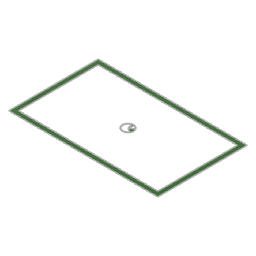
_car box.42bf6e30-fc25-4c0d-9044-dd2759e64512 (Autodesk Fusion 360 design; units mm, degrees)
Autodesk Fusion 360 part; units mm, degrees
sketch "Sketch1" plane through (0, 0, 0) normal (0, 0, 1) x (1, 0, 0)
  line L0 (-177.8, 101.6) -> (177.8, 101.6)
  line L1 (177.8, 101.6) -> (177.8, -101.6)
  line L2 (177.8, -101.6) -> (-177.8, -101.6)
  line L3 (-177.8, -101.6) -> (-177.8, 101.6)
  line L4 (-177.8, 101.6) -> (177.8, -101.6) construction
  line L5 (177.8, 101.6) -> (-177.8, -101.6) construction
  circle A0 centre (0, 0) radius 12.7
  line L6 (11.0267, -6.301) -> (10.7347, -6.1341)
  line L7 (0, 0) -> (11.0267, -6.301)
  line L8 (0, 0) -> (11.0267, 6.301)
  line L9 (-3.2992, 12.264) -> (0, 0)
  line L10 (3.2992, 12.264) -> (2.725, 12.1095)
  line L11 (2.725, 12.1095) -> (0, 0)
  circle A1 centre (0, 0) radius 14.3684
  line L12 (190.5, -114.3) -> (-190.5, -114.3)
  line L13 (-190.5, -114.3) -> (-190.5, 114.3)
  line L14 (-190.5, 114.3) -> (190.5, 114.3)
  line L15 (190.5, 114.3) -> (190.5, -114.3)
  dimension "d1" = 355.6
  dimension "d2" = 203.2
  dimension "d3" = -12.7
  constraint horizontal L0
  constraint perpendicular L0 L1
  constraint parallel L0 L2
  constraint parallel L1 L3
  constraint coincident L4 A0.centre
  constraint coincident L5 A0.centre
  constraint coincident A0.centre L7.start
  constraint coincident A0 L6.start
  constraint coincident L4 L6.start
  constraint coincident L4 L6.end
  constraint parallel L6 L7
  constraint coincident A0 L8.end
  constraint coincident L5 L8.end
  constraint coincident A0 L9.start
  constraint coincident A0 L10.start
  constraint perpendicular L9 L10
  measures "d1" distance of L1.end L2.end
  measures "d2" distance of L0.end L1.end
extrude "Extrude1" add sketch "Sketch1" along normal blind 0.254 contours A0 L6 L7 L8 | A0 L9 L10 L11 | A1 | L12 L13 L14 L15 makes body 1 at (8.465, -2.1003, 0) makes body 2 at (-59.2667, -110.0667, 0)
